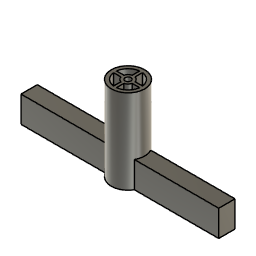
silnik góra v2 (Autodesk Fusion 360 design; units mm, degrees)
Autodesk Fusion 360 part; units mm, degrees
sketch "Szkic1" plane through (0, 0, 0) normal (0, 0, 1) x (1, 0, 0)
  line L0 (-100, 20.4) -> (-32, 20.4)
  line L1 (-32, 20.4) -> (-32, 14.8)
  line L2 (-32, 14.8) -> (-100, 14.8)
  line L3 (-100, 14.8) -> (-100, 20.4)
  line L4 (-98, 18.4) -> (-34, 18.4)
  line L5 (-34, 18.4) -> (-34, 16.8)
  line L6 (-34, 16.8) -> (-98, 16.8)
  line L7 (-98, 16.8) -> (-98, 18.4)
  line L8 (-71, 16.8) -> (-61, 16.8)
  line L9 (-61, 18.4) -> (-71, 18.4)
  line L10 (-71, 16.8) -> (-61, 16.8)
  line L11 (-61, 16.8) -> (-61, 14.8)
  line L12 (-61, 14.8) -> (-71, 14.8)
  line L13 (-71, 14.8) -> (-71, 16.8)
  dimension "d1" = 5.6
  dimension "d2" = 68
  dimension "d3" = 2
  dimension "d4" = 64
  dimension "d5" = 2
  dimension "d6" = 1.6
  constraint horizontal L0
  constraint vertical L1
  constraint horizontal L2
  constraint vertical L3
  constraint horizontal L4
  constraint vertical L5
  constraint horizontal L6
  constraint vertical L7
  constraint horizontal L8
  constraint horizontal L9
  constraint coincident L4 L9.start
  constraint coincident L6 L8.start
  constraint horizontal L10
  constraint vertical L11
  constraint horizontal L12
  constraint vertical L13
  constraint coincident L2 L11.end
  measures "d1" distance of L0.start L2.end
  measures "d2" distance of L0.start L0.end
  measures "d3" distance of L3 L7
  measures "d4" distance of L4.start L4.end
  measures "d5" distance of L2 L6
  measures "d6" distance of L4.end L5.end
extrude "Wyciągnięcie proste1" add sketch "Szkic1" along normal blind 9 contours L0 L1 L2 L3 L4 L5 L6 L7 L9 L11 L13
extrude "Wyciągnięcie proste2" add sketch "Szkic1" against normal blind 2 from surface at 9 contours L4 L5 L6 L7 L8 L9 L10
sketch "Szkic2" plane through (0, 0, 9) normal (0, 0, 1) x (-1, 0, 0)
  line L0 (100, -14.8) -> (71, -14.8)
  line L1 (71, -14.8) -> (71, -16.8)
  line L2 (71, -16.8) -> (61, -16.8)
  line L3 (61, -16.8) -> (61, -14.8)
  line L4 (61, -14.8) -> (32, -14.8)
  line L5 (32, -14.8) -> (32, -20.4)
  line L6 (32, -20.4) -> (100, -20.4)
  line L7 (100, -20.4) -> (100, -14.8)
  circle A0 centre (66, -17.6) radius 2.8
  circle A1 centre (66, -17.6) radius 1
  circle A2 centre (66, -17.6) radius 1.5
  circle A3 centre (66, -17.6) radius 2.1
  line L8 (66.6624, -16.2542) -> (66.6624, -15.6072)
  line L9 (65.3376, -16.2542) -> (65.3376, -15.6072)
  dimension "d14" = 5.6
  dimension "d15" = 2.8
  dimension "d16" = 2
  dimension "d17" = 3
  dimension "d18" = 4.2
  constraint concentric A0 A1
  constraint concentric A1 A2
  constraint concentric A2 A3
  constraint coincident A2 L8.start
  constraint coincident A3 L8.end
  constraint vertical L8
  constraint coincident A2 L9.start
  constraint coincident A3 L9.end
  constraint parallel L8 L9
  measures "d14" diameter of A0
  measures "d15" distance of L6 A0.centre
  measures "d16" diameter of A1
  measures "d17" diameter of A2
  measures "d18" diameter of A3
extrude "Wyciągnięcie proste3" add 1 faces at (-64.3333, 16.8, 7.6667) along direction (0, -1, 0) blind 2
move_body "Przesuń1" bodies 1 to x (1, 0, 0) y (0, 1, 0) z (0, 0, 1) at (66, -17.6, -9)
sketch "Szkic4" plane through (0, 0, 0) normal (0, 0, 1) x (-1, 0, 0)
  line L0 (34, 2.8) -> (-34, 2.8)
  line L1 (-34, 2.8) -> (-34, -2.8)
  line L2 (-34, -2.8) -> (34, -2.8)
  line L3 (34, -2.8) -> (34, 2.8)
  circle A0 centre (0, 0) radius 5.7306
  circle A1 centre (0, 0) radius 1
  circle A2 centre (0, 0) radius 2
  circle A3 centre (0, 0) radius 4.5
  line L4 (0.5, -4.7) -> (-0.5, -4.7)
  line L5 (-0.5, -4.7) -> (-0.5, -1.8)
  line L6 (-0.5, -1.8) -> (0.5, -1.8)
  line L7 (0.5, -1.8) -> (0.5, -4.7)
  line L8 (1.5, -0.5) -> (5, -0.5)
  line L9 (5, -0.5) -> (5, 0.5)
  line L10 (5, 0.5) -> (1.5, 0.5)
  line L11 (1.5, 0.5) -> (1.5, -0.5)
  line L12 (-1.5, -0.5) -> (-4.9, -0.5)
  line L13 (-4.9, -0.5) -> (-4.9, 0.5)
  line L14 (-4.9, 0.5) -> (-1.5, 0.5)
  line L15 (-1.5, 0.5) -> (-1.5, -0.5)
  line L16 (0.5, 1.5) -> (-0.5, 1.5)
  line L17 (-0.5, 1.5) -> (-0.5, 4.7)
  line L18 (-0.5, 4.7) -> (0.5, 4.7)
  line L19 (0.5, 4.7) -> (0.5, 1.5)
  dimension "d21" = 2
  constraint coincident A0.centre A1.centre
  constraint concentric A0 A1
  constraint concentric A0 A3
  constraint horizontal L4
  constraint vertical L5
  constraint horizontal L6
  constraint vertical L7
  constraint horizontal L8
  constraint vertical L9
  constraint horizontal L10
  constraint vertical L11
  constraint horizontal L12
  constraint vertical L13
  constraint horizontal L14
  constraint vertical L15
  constraint horizontal L16
  constraint vertical L17
  constraint horizontal L18
  constraint vertical L19
  measures "d21" diameter of A1
extrude "Wyciągnięcie proste4" add sketch "Szkic4" along normal blind -2 and the other way blind 0 contours L0 A2 L17 L19 | L0 A3 L17 L19 | L2 A3 L5 L7 | L2 A2 L5 L7
extrude "Wyciągnięcie proste5" add sketch "Szkic4" along normal blind 7 and the other way blind 9 contours L0 L2 A0 A3 L8 L9 L10 | L0 A0 A3 L17 L18 L19 | L0 L2 A0 A3 L12 L13 L14 | L2 A0 A3 L4 L5 L7 | A3 L8 L9 L10 | A3 L17 L18 L19 | A3 L12 L13 L14 | A3 L4 L5 L7
extrude "Wyciągnięcie proste6" add sketch "Szkic4" along normal blind 7 contours A2 L16 L17 L19 | A2 L5 L6 L7 L8 L10 L11 L12 L14 L15 L16 L17 L19 | A2 L8 L10 L11 | A2 L12 L14 L15 | A2 L5 L6 L7
extrude "Wyciągnięcie proste7" add sketch "Szkic4" along normal blind 7 contours L0 A2 L17 L19 | L0 A3 L17 L19 | A2 A3 L8 L10 | A2 A3 L12 L14 | L2 A3 L5 L7 | L2 A2 L5 L7
sketch "Szkic5" plane through (0, 0, -9) normal (0, 0, -1) x (1, 0, 0)
  line L0 (-3.5228, -2.8) -> (3.5228, -2.8)
  arc A0 (-3.5228, -2.8) -> (3.5228, -2.8) centre (0, 0) ccw
  arc A1 (-5, -2.8) -> (5, -2.8) centre (0, 0) ccw
  line L1 (5, -2.8) -> (34, -2.8)
  line L2 (34, -2.8) -> (34, 2.8)
  line L3 (34, 2.8) -> (5, 2.8)
  arc A2 (5, 2.8) -> (-5, 2.8) centre (0, 0) ccw
  line L4 (-5, 2.8) -> (-34, 2.8)
  line L5 (-34, 2.8) -> (-34, -2.8)
  line L6 (-34, -2.8) -> (-5, -2.8)
  arc A3 (-5.6745, 0.8) -> (-5.6745, -0.8) centre (0, 0) ccw
  line L7 (-5.6745, -0.8) -> (-32, -0.8)
  line L8 (-32, -0.8) -> (-32, 0.8)
  line L9 (-32, 0.8) -> (-5.6745, 0.8)
  arc A4 (4.4283, -0.8) -> (-4.4283, -0.8) centre (0, 0) ccw
  line L10 (4.4283, -0.8) -> (-4.4283, -0.8)
  arc A5 (5.6745, -0.8) -> (5.6745, 0.8) centre (0, 0) ccw
  line L11 (5.6745, 0.8) -> (32, 0.8)
  line L12 (32, 0.8) -> (32, -0.8)
  line L13 (32, -0.8) -> (5.6745, -0.8)
  line L14 (-32, 0.8) -> (32, 0.8)
  line L15 (32, 0.8) -> (32, -0.8)
  line L16 (32, -0.8) -> (-32, -0.8)
  line L17 (-32, -0.8) -> (-32, 0.8)
  constraint horizontal L14
  constraint vertical L15
  constraint horizontal L16
  constraint vertical L17
  constraint coincident L12.end L13.start
  constraint coincident L8.end L9.start
extrude "Wyciągnięcie proste8" cut sketch "Szkic5" against normal blind 7 contours A3 A4 L14 L16 | A4 A5 L14 L16
extrude "Wyciągnięcie proste9" add 1 faces at (-0.1667, 3.6269, 7) along direction (0, 0, 1) blind 13
equation "d1 = 2 mm + 2 mm + 1.6 mm"
equation "d2 = 64 mm + 4 mm"
equation "d15 = ( 5.6 / 2 ) * 1 mm"
